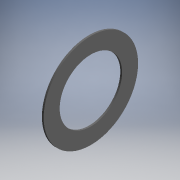
# Autodesk Inventor part: MR126ZZ Shield2
Saved by Autodesk Inventor 2017.3 (Build 213256000, 256)
## iProperties
Part Number: MR126ZZ Shield2
Material: Generic
Catalog Web Link: www.cadenas.de
Description: shielde_type_zz_zzs_S2-
Vendor: NSK_RB
Document SubType Name: Modeling
Designer: partserver
Manufacturer: NSK_RB
Mass: 0.0104775 g
Surface Area: 1.16523 cm^2
Volume: 0.0104775 cm^3
Density: 1 g/cm^3
Appearance: PSOLRGB-128-128-128
Category: PARTsolutions
Company: NSK_RB
Title: MR126ZZ Shield2
Author: Cadenas PARTsolutions
PSOL_IDENT_0: {$CADENAS_DATA\23d-libs\nsk_rb\roller_bearings\deep_groove_bb\exstra_small_miniatur_bb\metric_design
PSOL_IDENT_1: \shielded_type_zz_zzs_s2.prj},187 {VTYP=3D},{NB=MR126ZZ Shield2},{LINA=MR126ZZ Shield2},{NN=shielde_
PSOL_IDENT_2: type_zz_zzs_S2},{DATE=16.07.2021 00:25:30},{GEOMDATE=04.01.2008 00:00:00},{VERSION=},{LINEID=590},{W
PSOL_IDENT_3: BVAR=},{WBNUMERIC=}  {NB=MR126ZZ Shield2},{LINA=MR126ZZ Shield2},{KT=DUMMY},{IDNR=},{STAN=Standard},
PSOL_IDENT_4: {ORDER=MR126ZZ},{SD=6.0},{X=6.0},{DI1=7.73},{DI2=7.20},{SDE1=10.19},{SDE2=10.90},{D=12},{DD=12},{B=0
PSOL_IDENT_5: .0},{B1=4.0},{R=0.00},{R1=0.15},{CR1=715},{COR1=292},{CR2=73},{COR2=30.0},{LG=43000},{LO=50000},{DA=
PSOL_IDENT_6: 0.0},{DB=7.2},{DA1=0.0},{DB1=10.9},{RA=0.00},{RB=0.15},{MASS=1.74},{SC=1}
NB: MR126ZZ Shield2
NN: shielde_type_zz_zzs_S2
NBSYN: $ORDER. Shield2
LINA: MR126ZZ Shield2
CATALOG: NSK Rolling Bearing
STAN: Standard
ORDER: MR126ZZ
SD: 6
X: 6
DI1: 7.73
DI2: 7.2
SDE1: 10.19
SDE2: 10.9
D: 12
DD: 12
B: 0
B1: 4
R: 0
R1: 0.15
CR1: 715
COR1: 292
CR2: 73
COR2: 30
LG: 43000
LO: 50000
DA: 0
DB: 7.2
DA1: 0
DB1: 10.9
RA: 0
RB: 0.15
MASS: 1.74
SC: 1
SUPPLIER: NSK_RB
ARTICLENO: MR126ZZ Shield2
BOMINFO: MR126ZZ Shield2
CREATOR: CADENAS GmbH
Autodesk Inventor part; units mm, degrees
sketch "Sketch_1" plane through (0, 0, 0) normal (0, 0, 1) x (1, 0, 0)
  line L0 (3.9336, 0) -> (3.7344, 0)
  line L1 (3.7344, 3.6) -> (3.9336, 3.6)
  line L2 (3.9336, 3.6) -> (3.9336, 5.45)
  line L3 (3.9336, 5.45) -> (3.7344, 5.45)
  line L4 (3.7344, 5.45) -> (3.7344, 3.6)
  constraints: 10 end point
revolve "Revolution1" add sketch "Sketch_1" angle 360 about axis through (3.9336, 0, 0) along (1, 0, 0)
ref_plane "ip_st_s2_XY" through (3.7344, 0, 0) normal (1, 0, 0) x (0, 0, -1)
ref_plane "ip_st_s2_YZ" through (3.7344, 0, 0) normal (0, 0, -1) x (0, 1, 0)
ref_plane "ip_st_s2_ZX" through (3.7344, 0, 0) normal (0, 1, 0) x (1, 0, 0)
body "Solid1"
